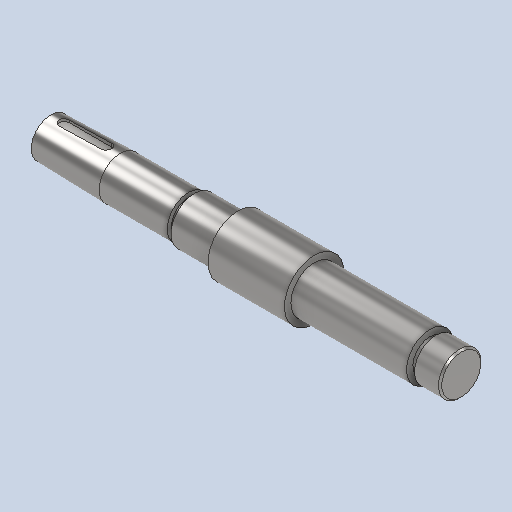
# Autodesk Inventor part: Вал
Saved by Autodesk Inventor 2022.1 (Build 261234020, 234B)
## iProperties
CustomPartVersion: 1
Created: 2021-09-09
Part Number: Вал
Material: Сталь, углеродистая
Document SubType Name: Modeling
Designer: Dison
Density: 1 g/cm^3
Appearance: С умеренной полировкой
Length: 483,000 мм
Author: Dison
Autodesk Inventor part; units mm, degrees
ref_plane "Начальная плоскость" through (0, 0, 0) normal (1, 0, 0) x (0, 1, 0)
ref_plane "XY Plane" through (0, 0, 0) normal (0, 0, 1) x (1, 0, 0)
sketch "Основной эскиз" plane through (0, 0, 0) normal (0, 0, 1) x (1, 0, 0)
  line L0 (0, 0) -> (483, 0)
  line L1 (0, 0) -> (0, 22.95)
  line L2 (0, 22.95) -> (82, 25)
  line L3 (162, 25) -> (162, 20)
  line L4 (82, 25) -> (162, 25)
  line L5 (162, 20) -> (169, 20)
  line L6 (169, 20) -> (169, 27.5)
  line L7 (169, 27.5) -> (220, 27.5)
  line L8 (220, 27.5) -> (220, 35)
  line L9 (310, 35) -> (310, 27.5)
  line L10 (220, 35) -> (310, 35)
  line L11 (446, 27.5) -> (446, 20)
  line L12 (310, 27.5) -> (446, 27.5)
  line L13 (446, 20) -> (453, 20)
  line L14 (453, 20) -> (453, 25)
  line L15 (483, 25) -> (483, 0)
  line L16 (453, 25) -> (483, 25)
  dimension "d3" = 50
  dimension "d4" = 40
  dimension "d5" = 55
  dimension "d6" = 70
  dimension "d7" = 55
  dimension "d8" = 40
  dimension "d9" = 50
  constraints: 34 end point, 8 vertical, 2 horizontal
  measures "d3" diameter of L4 L0
  measures "d4" diameter of L5 L0
  measures "d5" diameter of L7 L0
  measures "d6" diameter of L10 L0
  measures "d7" diameter of L12 L0
  measures "d8" diameter of L13 L0
  measures "d9" diameter of L16 L0
revolve "Вращение1" add sketch "Основной эскиз" angle 360 about axis through (0, 0, 0) along (1, 0, 0)
chamfer "Фаска1" distance 2 angle 45 1 edges at (483, -25, 0) measured on face at (463, 24.6763, -4.0103)
ref_plane "РабПлоскость1" through (0, 25, 0) normal (0, 1, 0) x (-1, 0, 0)
sketch "Эскиз3" plane through (0, 25, 0) normal (0, 1, 0) x (-1, 0, 0)
  line L0 (-16, 0) -> (-66, 0) construction
  line L1 (-16, 6) -> (-66, 6)
  line L2 (-66, -6) -> (-16, -6)
  arc A0 (-16, -6) -> (-16, 6) centre (-16, 0) ccw
  arc A1 (-66, 6) -> (-66, -6) centre (-66, 0) ccw
  line L3 (0, -22.95) -> (0, 22.95) projected
  line L4 (14.4, 0) -> (-86.4, 0) projected
  point P0 (0, 0)
  point P1 (-41, 0)
  dimension "d15" = 25
  dimension "d16" = 12
  dimension "d17" = 41
  constraints: 8 end point, 4 point on circle, 4 tangent, 2 centre point, 1 horizontal, 1 midpoint, 1 parallel, 1 point on line
  measures "d15" distance of point (-41, 0) L0.end
  measures "d16" diameter of A1
  measures "d17" distance of point (0, 0) point (-41, 0)
extrude "Выдавливание1" cut sketch "Эскиз3" against normal blind 5
equation "\"Length\" = 483"
